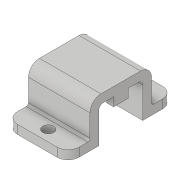
# Autodesk Inventor part: MotorCap
Saved by Autodesk Inventor 2017 (Build 210142000, 142)
## iProperties
Created: 2019-06-11
Part Number: MotorCap
Material: Generic
Document SubType Name: Modeling
Designer: markg
Density: 1 g/cm^3
Appearance: Default
Author: markg
Autodesk Inventor part; units mm, degrees
ref_plane "YZ Plane" through (0, 0, 0) normal (1, 0, 0) x (0, 1, 0)
ref_plane "XZ Plane" through (0, 0, 0) normal (0, 1, 0) x (-1, 0, 0)
ref_plane "XY Plane" through (0, 0, 0) normal (0, 0, 1) x (1, 0, 0)
sketch "Sketch1" plane through (0, 0, 0) normal (1, 0, 0) x (0, 1, 0)
  line L0 (0, 15.24) -> (2.54, 15.24)
  line L1 (2.54, 15.24) -> (2.54, 8.89)
  line L2 (2.54, 8.89) -> (12.7, 8.89)
  line L3 (12.7, 8.89) -> (12.7, -8.89)
  line L4 (12.7, -8.89) -> (2.54, -8.89)
  line L5 (2.54, -8.89) -> (2.54, -15.24)
  line L6 (0, 15.24) -> (0, 6.35)
  line L7 (0, 6.35) -> (10.16, 6.35)
  line L8 (10.16, 6.35) -> (10.16, -6.35)
  line L9 (10.16, -6.35) -> (0, -6.35)
  line L10 (0, -6.35) -> (0, -15.24)
  line L11 (0, -15.24) -> (2.54, -15.24)
  point P0 (0, 0)
  dimension "d0" = 12.7
  dimension "d1" = 10.16
  dimension "d2" = 12.7
  dimension "d3" = 17.78
  dimension "d4" = 2.54
  dimension "d5" = 6.35
  dimension "d6" = 2.54
  dimension "d7" = 8.89
  dimension "d8" = 8.89
  constraints: 24 end point, 8 perpendicular, 3 point on line, 2 vertical, 1 horizontal
  measures "d0" distance between parallel lines of L9 L7
  measures "d1" distance from line of L8 point (0, 0)
  measures "d2" distance from line of point (0, 0) L3
  measures "d3" distance of L2.end L3.end
  measures "d4" distance between parallel lines of L7 L2
  measures "d5" distance from line of L9 point (0, 0)
  measures "d6" distance of L0.start L0.end
  measures "d7" distance of L0.start L6.end
  measures "d8" distance of L9.end L10.end
extrude "Extrusion1" add sketch "Sketch1" along normal blind 17.78
sketch "Sketch2" plane through (0, 10.16, -6.35) normal (0, -1, 0) x (1, 0, 0)
  line L0 (17.78, 8.4328) -> (15.748, 8.4328)
  line L1 (15.748, 8.4328) -> (15.748, 4.2164)
  line L2 (15.748, 4.2164) -> (17.78, 4.2164)
  line L3 (17.78, 4.2164) -> (17.78, 8.4328)
  line L4 (17.78, 12.7) -> (17.78, 0) projected
  line L5 (0, 0) -> (17.78, 0) projected
  point P0 (0, 6.35)
  dimension "d11" = 2.032
  dimension "d12" = 0
  dimension "d13" = 4.2164
  dimension "d14" = 4.2164
  constraints: 8 end point, 2 parallel, 1 horizontal, 1 perpendicular
  measures "d11" distance of L2.end L1.end
  measures "d12" distance between parallel lines of L4 L3
  measures "d13" distance of L0.end L1.end
  measures "d14" distance between parallel lines of L5 L2
extrude "Extrusion2" add sketch "Sketch2" along normal blind 2.54
fillet "Fillet1" radius 1.27 2 edges at (8.89, 10.16, 6.35) (8.89, 10.16, -6.35)
fillet "Fillet2" radius 3.175 2 edges at (8.89, 12.7, 8.89) (8.89, 12.7, -8.89)
sketch "Sketch3" plane through (0, 2.54, 15.24) normal (0, 1, 0) x (1, 0, 0)
  circle A0 centre (8.89, 3.175) radius 1.5875
  circle A1 centre (8.89, 27.305) radius 1.5875
  line L0 (0, 24.13) -> (0, 30.48) projected
  line L1 (0, 0) -> (0, 6.35) projected
  line L2 (0, 0) -> (17.78, 0) projected
  line L3 (0, 30.48) -> (17.78, 30.48) projected
  point P0 (0, 15.24)
  dimension "d19" = 3.175
  dimension "d20" = 3.175
  dimension "d21" = 8.89
  dimension "d22" = 8.89
  dimension "d23" = 3.175
  dimension "d24" = 3.175
  constraints: 2 centre point
  measures "d19" diameter of A0
  measures "d20" diameter of A1
  measures "d21" distance from line of L0 A1.centre
  measures "d22" distance from line of A0.centre L1
  measures "d23" distance from line of L2 A0.centre
  measures "d24" distance from line of L3 A1.centre
fillet "Fillet3" radius 3.175 4 edges at (17.78, 1.27, 15.24) (17.78, 1.27, -15.24) (0, 1.27, -15.24) (0, 1.27, 15.24)
extrude "Extrusion3" cut sketch "Sketch3" against normal blind 6.985
fillet "Fillet4" radius 0.635 2 edges at (8.89, 2.54, 8.89) (8.89, 2.54, -8.89)
body "Solid1"
